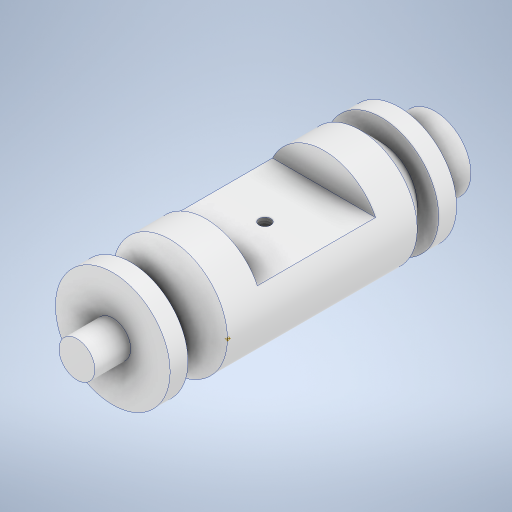
# Autodesk Inventor part: Part1
Saved by Autodesk Inventor 2024 (Build 280153000, 153)
## iProperties
Created: 2023-08-25
Part Number: Part1
Material: Aluminum 6061
Document SubType Name: Modeling
Designer: Nate
Density: 2.7 g/cm^3
Appearance: Aluminum - Flat
Mass: 150.347 g
Surface Area: 121.767 cm^2
Volume: 55.6841 cm^3
Author: Nate
Autodesk Inventor part; units mm, degrees
ref_plane "YZ Plane" through (0, 0, 0) normal (1, 0, 0) x (0, 1, 0)
ref_plane "XZ Plane" through (0, 0, 0) normal (0, 1, 0) x (-1, 0, 0)
ref_plane "XY Plane" through (0, 0, 0) normal (0, 0, 1) x (1, 0, 0)
sketch "Sketch2" plane through (0, 0, 0) normal (1, 0, 0) x (0, 1, 0)
  line L0 (0, 0) -> (7, 0)
  line L1 (0, 0) -> (16, 0)
  line L2 (10, -64) -> (10, -74)
  line L3 (10, -74) -> (0, -74)
  line L4 (0, -74) -> (0, -64)
  line L5 (0, 0) -> (16, 0)
  line L6 (0, 0) -> (16, 0)
  line L7 (16, 0) -> (16, 0)
  line L8 (5, 11) -> (0, 11)
  line L9 (0, 11) -> (0, 0)
  line L10 (0, 11) -> (16, 11)
  line L11 (16, 11) -> (16, 16)
  line L12 (16, 16) -> (0, 16)
  line L13 (0, 16) -> (0, 11)
  line L14 (16, 0) -> (5, 11)
  line L15 (0, 0) -> (16, 0)
  line L16 (16, 0) -> (16, -53)
  line L17 (10, -59) -> (0, -59)
  line L18 (0, -59) -> (0, 0)
  line L19 (0, -59) -> (16, -59)
  line L20 (16, -59) -> (16, -64)
  line L21 (16, -64) -> (0, -64)
  line L22 (0, -64) -> (0, -59)
  line L23 (10, -59) -> (16, -53)
  line L24 (0, 16) -> (5, 16)
  line L25 (5, 16) -> (5, 26)
  line L26 (5, 26) -> (0, 26)
  line L27 (0, 26) -> (0, 16)
  point P0 (8, -64)
  point P1 (8, 0)
  point P2 (8, 11)
  point P3 (8, 16)
  point P4 (5, -59)
  point P5 (5, -74)
  dimension "d7" = 10
  dimension "d14" = 16
  dimension "d15" = 11
  dimension "d18" = 16
  dimension "d19" = 59
  dimension "d24" = 5
  dimension "d26" = 5
  dimension "d27" = 10
  dimension "d45" = 53
  dimension "d46" = 5
  dimension "d47" = 10
  constraints: 56 end point, 11 parallel, 8 horizontal, 7 point on line, 5 midpoint, 5 perpendicular
  measures "d7" distance of L2.end L3.end
  measures "d14" distance of L8.end point (16, 11)
  measures "d15" distance of point (16, 11) L6.end
  measures "d18" distance of point (16, -59) L17.end
  measures "d19" distance of L15.end point (16, -59)
  measures "d24" distance of point (8, 11) point (8, 16)
  measures "d26" distance of L26.end L25.end
  measures "d27" distance of L25.end L24.end
  measures "d45" distance from line of L16.end L1
  measures "d46" distance from line of L21 point (5, -59)
  measures "d47" distance from line of point (5, -74) L21
revolve "Revolution1" add sketch "Sketch2" angle 360 about axis through (0, 0, -59) along (0, 0, 1)
sketch "Sketch5" plane through (0, 0, 0) normal (1, 0, 0) x (0, 1, 0)
  line L0 (7, -10) -> (16, -10)
  line L1 (16, -10) -> (16, -43)
  line L2 (16, -43) -> (7, -43)
  line L3 (7, -43) -> (7, -10)
  point P0 (0, 0)
  point P1 (11.5, -10)
  dimension "d28" = 9
  dimension "d29" = 33
  dimension "d30" = 10
  dimension "d31" = 7
  constraints: 8 end point, 2 parallel, 1 horizontal, 1 midpoint, 1 perpendicular
  measures "d28" distance of L1.end L2.end
  measures "d29" distance of L0.end L1.end
  measures "d30" vertical distance of point (11.5, -10) point (0, 0)
  measures "d31" distance from line of L3 point (0, 0)
extrude "Extrusion1" cut sketch "Sketch5" along normal through all both and the other way through all
sketch "Sketch6" plane through (-14.3875, 7, -10) normal (0, 1, 0) x (1, 0, 0)
  line L0 (0, 0) -> (0, 33) projected
  line L1 (0, 0) -> (28.775, 0) projected
  line L2 (28.775, 33) -> (28.775, 0) projected
  line L3 (28.775, 33) -> (0, 33) projected
  circle A0 centre (14.3875, 16.5) radius 2
  point P0 (14.3875, -10)
  dimension "d34" = 4
  constraints: 1 centre point
  measures "d34" diameter of A0
hole "Hole1" at (0, 7, -26.5) direction (0, -1, 0) diameter 3.242 end through all thread size "M4x0.7" class "6H" standard "ISO Metric profile"
move or copy body "Move Body1" bodies to move or copy 1 copy no translate (-16, 0, 0)
body "Solid1"
